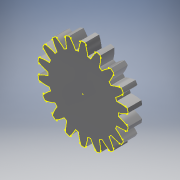
# Autodesk Inventor part: Цилиндрическое зубчатое зацепление1
Saved by Autodesk Inventor 2019 (Build 230136000, 136)
## iProperties
Created: 2020-02-27
Part Number: Цилиндрическое зубчатое зацепление1
Material: Steel
Document SubType Name: Modeling
Designer: Петров Иван
Categories: <?xml version="1.0" encoding="UTF-16"?> <MemberInstance><Categories><FamilyTemplate><FamilyTemplateParameter ValueType="xs:double" Id="1" ObjectReferenceKey="da_z" ObjectType="kUserParameterObject"/><FamilyTemplateParameter ValueType="xs:double" Id="2" ObjectReferenceKey="da_b" ObjectType="kUserParameterObject"/><FamilyTemplateParameter ValueType="xs:double" Id="3" ObjectReferenceKey="da_beta" ObjectType="kUserParameterObject"/><FamilyTemplateParameter ValueType="xs:double" Id="4" ObjectReferenceKey="da_da" ObjectType="kUserParameterObject"/><FamilyTemplateParameter ValueType="xs:double" Id="5" ObjectReferenceKey="da_aw" ObjectType="kUserParameterObject"/><FamilyTemplateParameter ValueType="xs:string" Id="6" ObjectReferenceKey="EAIAABAAAACIAQAAAAAAAIAAAAAAAAAA" ObjectType="83910656" SubObjectId="SurfaceGeometry"/></FamilyTemplate><ParamToTemplateMap><ParamToTemplate CategoryParameter="//CategoryParameter[@InternalName='046C89C9-8512-4d59-83FE-43B91F4F132A']" TemplateParameter="1"/><ParamToTemplate CategoryParameter="//CategoryParameter[@InternalName='2552DF32-E462-4b46-AEBF-C6C7768E72AC']" TemplateParameter="2"/><ParamToTemplate CategoryParameter="//CategoryParameter[@InternalName='C9EE641D-15FC-4fae-A226-E94C4372FDD7']" TemplateParameter="3"/><ParamToTemplate><ParamToTemplate CategoryParameter="//CategoryParameter[@InternalName='00B6519A-459B-49c7-AD84-2E56D39A5744']" ConstantValue="0.000000"/></ParamToTemplate><ParamToTemplate><ParamToTemplate CategoryParameter="//CategoryParameter[@InternalName='04B31F0E-C7A6-4894-AA32-9629BEFACF47']" ConstantValue="1.000000"/></ParamToTemplate><ParamToTemplate><ParamToTemplate CategoryParameter="//CategoryParameter[@InternalName='43CBEC2E-7847-49e7-A936-2F7889FCB2D9']" ConstantValue="0.250000"/></ParamToTemplate><ParamToTemplate><ParamToTemplate CategoryParameter="//CategoryParameter[@InternalName='B1EFC894-105D-4ebd-86BF-FA20ED196853']" ConstantValue="0.350000"/></ParamToTemplate><ParamToTemplate><ParamToTemplate CategoryParameter="//CategoryParameter[@InternalName='51175063-3D10-4879-93E8-6246FE8B403D']" ConstantValue="2060000000.000000"/></ParamToTemplate><ParamToTemplate><ParamToTemplate CategoryParameter="//CategoryParameter[@InternalName='A3A52E27-4454-46a9-B0BD-C932399B70AF']" ConstantValue="0.300000"/></ParamToTemplate><ParamToTemplate><ParamToTemplate CategoryParameter="//CategoryParameter[@InternalName='91B76062-C214-41d9-B1B9-14D2AB99603D']" ConstantValue="0.225000"/></ParamToTemplate><ParamToTemplate><ParamToTemplate CategoryParameter="//CategoryParameter[@InternalName='374E806E-8B8A-4dda-A9AA-1039D6500AD2']" ConstantValue="4.444444"/></ParamToTemplate><ParamToTemplate><ParamToTemplate CategoryParameter="//CategoryParameter[@InternalName='2D373A89-B862-43d6-8D0B-0CBF12AB9F6C']" ConstantValue="0.523599"/></ParamToTemplate><ParamToTemplate CategoryParameter="//CategoryParameter[@InternalName='37777632-D6A2-4fac-9D53-DB8ACD95C989']" TemplateParameter="4"/><ParamToTemplate CategoryParameter="//CategoryParameter[@InternalName='FD1017F1-B727-4f7e-9707-0F86F1FF9423']" TemplateParameter="5"/><ParamToTemplate><ParamToTemplate CategoryParameter="//CategoryParameter[@InternalName='9E1B4470-B2D3-4ff1-B813-535BB4CDF51A']" ConstantValue="3520000.000000"/></ParamToTemplate><ParamToTemplate><ParamToTemplate CategoryParameter="//CategoryParameter[@InternalName='F8452263-BFF6-458c-9FB1-07C4B99E95CD']" ConstantValue="11400000.000000"/></ParamToTemplate><ParamToTemplate><ParamToTemplate CategoryParameter="//CategoryParameter[@InternalName='3E3BB259-FD49-497f-8171-6EBC954A3479']" ConstantValue="2.000000"/></ParamToTemplate><ParamToTemplate CategoryParameter="//CategoryParameter[@InternalName='27C3BAF2-7550-4e4b-AE2C-0DB134B7D9B7']" TemplateParameter="6"/></ParamToTemplateMap><Category DisplayName="Gear" InternalName="DC85795E-93AB-48d5-8EEE-5A27447B64BD" Mnemonic="Gear"><CategoryParameter DisplayName="z" InternalName="046C89C9-8512-4d59-83FE-43B91F4F132A" Mnemonic="z"/><CategoryParameter DisplayName="b" InternalName="2552DF32-E462-4b46-AEBF-C6C7768E72AC" Mnemonic="b"/><CategoryParameter DisplayName="||b|" InternalName="C9EE641D-15FC-4fae-A226-E94C4372FDD7" Mnemonic="beta"/><CategoryParameter DisplayName="x" InternalName="00B6519A-459B-49c7-AD84-2E56D39A5744" Mnemonic="x"/><CategoryParameter DisplayName="a*" InternalName="04B31F0E-C7A6-4894-AA32-9629BEFACF47" Mnemonic="a"/><CategoryParameter DisplayName="c*" InternalName="43CBEC2E-7847-49e7-A936-2F7889FCB2D9" Mnemonic="c"/><CategoryParameter DisplayName="r|.f|*" InternalName="B1EFC894-105D-4ebd-86BF-FA20ED196853" Mnemonic="rf"/><CategoryParameter DisplayName="E" InternalName="51175063-3D10-4879-93E8-6246FE8B403D" Mnemonic="E"/><CategoryParameter DisplayName="||m|" InternalName="A3A52E27-4454-46a9-B0BD-C932399B70AF" Mnemonic="mi"/><Category DisplayName="SpurGear" InternalName="26C5A22E-A91E-4dfd-A3B3-23CCAFAE1764" Mnemonic="SpurGear"><CategoryParameter DisplayName="m" InternalName="91B76062-C214-41d9-B1B9-14D2AB99603D" Mnemonic="m"/><CategoryParameter DisplayName="P" InternalName="374E806E-8B8A-4dda-A9AA-1039D6500AD2" Mnemonic="PP"/><CategoryParameter DisplayName="||a|" InternalName="2D373A89-B862-43d6-8D0B-0CBF12AB9F6C" Mnemonic="alpha"/><CategoryParameter DisplayName="d|.a|" InternalName="37777632-D6A2-4fac-9D53-DB8ACD95C989" Mnemonic="da"/><CategoryParameter DisplayName="a|.w|" InternalName="FD1017F1-B727-4f7e-9707-0F86F1FF9423" Mnemonic="aw"/><CategoryParameter DisplayName="||s||.Flim|" InternalName="9E1B4470-B2D3-4ff1-B813-535BB4CDF51A" Mnemonic="sFlim"/><CategoryParameter DisplayName="||s||.Hlim|" InternalName="F8452263-BFF6-458c-9FB1-07C4B99E95CD" Mnemonic="sHlim"/><CategoryParameter DisplayName="тип" InternalName="3E3BB259-FD49-497f-8171-6EBC954A3479" Mnemonic="type"/><CategoryParameter DisplayName="PitchDiameter" InternalName="27C3BAF2-7550-4e4b-AE2C-0DB134B7D9B7" Mnemonic="IDS_PITCHDIAM"/></Category></Category></Categories></MemberInstance>
Density: 1 g/cm^3
Appearance: Steel
CustomPartVersion: 1
Author: Петров Иван
Autodesk Inventor part; units mm, degrees
ref_plane "YZ Plane" through (0, 0, 0) normal (1, 0, 0) x (0, 1, 0)
ref_plane "XZ Plane" through (0, 0, 0) normal (0, 1, 0) x (-1, 0, 0)
ref_plane "XY Plane" through (0, 0, 0) normal (0, 0, 1) x (1, 0, 0)
sketch "Sketch1" plane through (0, 0, 0) normal (0, 0, 1) x (1, 0, 0)
  circle A0 centre (0, 0) radius 22.4858
  dimension "d0" = 44.9715
  constraints: 1 centre point
  measures "d0" diameter of A0
extrude "Extrusion1" add sketch "Sketch1" along normal blind 7
ref_plane "Work Plane2" through (0, 0, 3.5) normal (0, 0, 1) x (1, 0, 0)
sketch "Sketch2" plane through (0, 0, 0) normal (0, 0, -1) x (-1, 0, 0)
  circle A0 centre (0, 0) radius 22.4858 projected
  circle A1 centre (0, 0) radius 20
  dimension "d3" = 40
  constraints: 1 centre point, 1 coincident
  measures "d3" diameter of A1
surface extrude "Средний диаметр" sketch "Sketch2" against normal through all shown no curves A1
ref_plane "Work Plane8" through (0, 0, 0) normal (0.9848078, 0.1736482, 0) x (0, 0, 1)
ref_plane "Work Plane9" through (0, 0, 0) normal (1, 0, 0) x (0, 1, 0)
spur gear teeth "Цилиндрическое зубчатое зацепление" teeth 18 pitch diameter 40.5 tip diameter 44.9715 root diameter 34.875 face width 7 start plane through (0, 0, 0) normal (0, 0, -1) x (-1, 0, 0)
sketch "Эскиз3" plane through (0, 0, 7) normal (0, 0, 1) x (1, 0, 0)
  arc A0 (-8.6049, 20.7741) -> (-8.0517, 15.4673) centre (8.9595, 19.9228) ccw projected
  arc A1 (-8.0517, 15.4673) -> (-9.3692, 14.7066) centre (0, 0) ccw projected
  arc A2 (-9.3692, 14.7066) -> (-13.6885, 17.8391) centre (-21.7334, 2.2022) ccw projected
  arc A3 (-13.6885, 17.8391) -> (-15.1912, 16.5782) centre (0, 0) ccw projected
  arc A4 (-15.1912, 16.5782) -> (-12.8563, 11.7806) centre (1.6052, 21.7856) ccw projected
  arc A5 (-12.8563, 11.7806) -> (-13.8341, 10.6153) centre (0, 0) ccw projected
  arc A6 (-13.8341, 10.6153) -> (-18.9643, 12.0816) centre (-21.1759, -5.3638) ccw projected
  arc A7 (-18.9643, 12.0816) -> (-19.9451, 10.3828) centre (0, 0) ccw projected
  arc A8 (-19.9451, 10.3828) -> (-16.1101, 6.673) centre (-5.9427, 21.0208) ccw projected
  arc A9 (-16.1101, 6.673) -> (-16.6304, 5.2436) centre (0, 0) ccw projected
  arc A10 (-16.6304, 5.2436) -> (-21.9528, 4.8668) centre (-18.0643, -12.2829) ccw projected
  arc A11 (-21.9528, 4.8668) -> (-22.2934, 2.935) centre (0, 0) ccw projected
  arc A12 (-22.2934, 2.935) -> (-17.4209, 0.7606) centre (-12.7739, 17.7205) ccw projected
  arc A13 (-17.4209, 0.7606) -> (-17.4209, -0.7606) centre (0, 0) ccw projected
  arc A14 (-17.4209, -0.7606) -> (-22.2934, -2.935) centre (-12.7739, -17.7205) ccw projected
  arc A15 (-22.2934, -2.935) -> (-21.9528, -4.8668) centre (0, 0) ccw projected
  arc A16 (-21.9528, -4.8668) -> (-16.6304, -5.2436) centre (-18.0643, 12.2829) ccw projected
  arc A17 (-16.6304, -5.2436) -> (-16.1101, -6.673) centre (0, 0) ccw projected
  arc A18 (-16.1101, -6.673) -> (-19.9451, -10.3828) centre (-5.9427, -21.0208) ccw projected
  arc A19 (-19.9451, -10.3828) -> (-18.9643, -12.0816) centre (0, 0) ccw projected
  arc A20 (-18.9643, -12.0816) -> (-13.8341, -10.6153) centre (-21.1759, 5.3638) ccw projected
  arc A21 (-13.8341, -10.6153) -> (-12.8563, -11.7806) centre (0, 0) ccw projected
  arc A22 (-12.8563, -11.7806) -> (-15.1912, -16.5782) centre (1.6052, -21.7856) ccw projected
  arc A23 (-15.1912, -16.5782) -> (-13.6885, -17.8391) centre (0, 0) ccw projected
  arc A24 (-13.6885, -17.8391) -> (-9.3692, -14.7066) centre (-21.7334, -2.2022) ccw projected
  arc A25 (-9.3692, -14.7066) -> (-8.0517, -15.4673) centre (0, 0) ccw projected
  arc A26 (-8.0517, -15.4673) -> (-8.6049, -20.7741) centre (8.9595, -19.9228) ccw projected
  arc A27 (-8.6049, -20.7741) -> (-6.7616, -21.445) centre (0, 0) ccw projected
  arc A28 (-6.7616, -21.445) -> (-3.7742, -17.0242) centre (-19.6695, -9.5027) ccw projected
  arc A29 (-3.7742, -17.0242) -> (-2.2761, -17.2883) centre (0, 0) ccw projected
  arc A30 (-2.2761, -17.2883) -> (-0.9808, -22.4644) centre (15.2332, -15.6569) ccw projected
  arc A31 (-0.9808, -22.4644) -> (0.9808, -22.4644) centre (0, 0) ccw projected
  arc A32 (0.9808, -22.4644) -> (2.2761, -17.2883) centre (-15.2332, -15.6569) ccw projected
  arc A33 (2.2761, -17.2883) -> (3.7742, -17.0242) centre (0, 0) ccw projected
  arc A34 (3.7742, -17.0242) -> (6.7616, -21.445) centre (19.6695, -9.5027) ccw projected
  arc A35 (6.7616, -21.445) -> (8.6049, -20.7741) centre (0, 0) ccw projected
  arc A36 (8.6049, -20.7741) -> (8.0517, -15.4673) centre (-8.9595, -19.9228) ccw projected
  arc A37 (8.0517, -15.4673) -> (9.3692, -14.7066) centre (0, 0) ccw projected
  arc A38 (9.3692, -14.7066) -> (13.6885, -17.8391) centre (21.7334, -2.2022) ccw projected
  arc A39 (13.6885, -17.8391) -> (15.1912, -16.5782) centre (0, 0) ccw projected
  arc A40 (15.1912, -16.5782) -> (12.8563, -11.7806) centre (-1.6052, -21.7856) ccw projected
  arc A41 (12.8563, -11.7806) -> (13.8341, -10.6153) centre (0, 0) ccw projected
  arc A42 (13.8341, -10.6153) -> (18.9643, -12.0816) centre (21.1759, 5.3638) ccw projected
  arc A43 (18.9643, -12.0816) -> (19.9451, -10.3828) centre (0, 0) ccw projected
  arc A44 (19.9451, -10.3828) -> (16.1101, -6.673) centre (5.9427, -21.0208) ccw projected
  arc A45 (16.1101, -6.673) -> (16.6304, -5.2436) centre (0, 0) ccw projected
  arc A46 (16.6304, -5.2436) -> (21.9528, -4.8668) centre (18.0643, 12.2829) ccw projected
  arc A47 (21.9528, -4.8668) -> (22.2934, -2.935) centre (0, 0) ccw projected
  arc A48 (22.2934, -2.935) -> (17.4209, -0.7606) centre (12.7739, -17.7205) ccw projected
  arc A49 (17.4209, -0.7606) -> (17.4209, 0.7606) centre (0, 0) ccw projected
  arc A50 (17.4209, 0.7606) -> (22.2934, 2.935) centre (12.7739, 17.7205) ccw projected
  arc A51 (22.2934, 2.935) -> (21.9528, 4.8668) centre (0, 0) ccw projected
  arc A52 (21.9528, 4.8668) -> (16.6304, 5.2436) centre (18.0643, -12.2829) ccw projected
  arc A53 (16.6304, 5.2436) -> (16.1101, 6.673) centre (0, 0) ccw projected
  arc A54 (16.1101, 6.673) -> (19.9451, 10.3828) centre (5.9427, 21.0208) ccw projected
  arc A55 (19.9451, 10.3828) -> (18.9643, 12.0816) centre (0, 0) ccw projected
  arc A56 (18.9643, 12.0816) -> (13.8341, 10.6153) centre (21.1759, -5.3638) ccw projected
  arc A57 (13.8341, 10.6153) -> (12.8563, 11.7806) centre (0, 0) ccw projected
  arc A58 (12.8563, 11.7806) -> (15.1912, 16.5782) centre (-1.6052, 21.7856) ccw projected
  arc A59 (15.1912, 16.5782) -> (13.6885, 17.8391) centre (0, 0) ccw projected
  arc A60 (13.6885, 17.8391) -> (9.3692, 14.7066) centre (21.7334, 2.2022) ccw projected
  arc A61 (9.3692, 14.7066) -> (8.0517, 15.4673) centre (0, 0) ccw projected
  arc A62 (8.0517, 15.4673) -> (8.6049, 20.7741) centre (-8.9595, 19.9228) ccw projected
  arc A63 (8.6049, 20.7741) -> (6.7616, 21.445) centre (0, 0) ccw projected
  arc A64 (6.7616, 21.445) -> (3.7742, 17.0242) centre (19.6695, 9.5027) ccw projected
  arc A65 (3.7742, 17.0242) -> (2.2761, 17.2883) centre (0, 0) ccw projected
  arc A66 (2.2761, 17.2883) -> (0.9808, 22.4644) centre (-15.2332, 15.6569) ccw projected
  arc A67 (0.9808, 22.4644) -> (-0.9808, 22.4644) centre (0, 0) ccw projected
  arc A68 (-0.9808, 22.4644) -> (-2.2761, 17.2883) centre (15.2332, 15.6569) ccw projected
  arc A69 (-2.2761, 17.2883) -> (-3.7742, 17.0242) centre (0, 0) ccw projected
  arc A70 (-3.7742, 17.0242) -> (-6.7616, 21.445) centre (-19.6695, 9.5027) ccw projected
  arc A71 (-6.7616, 21.445) -> (-8.6049, 20.7741) centre (0, 0) ccw projected
equation "\"d0\" = da_da"
equation "\"d1\" = da_b"
equation "\"d3\" = da_dw"
equation "\"da_da\" = 44.971512"
equation "\"da_b\" = 7"
equation "\"da_dw\" = 40"
body "Solid1"
body "Srf1"
